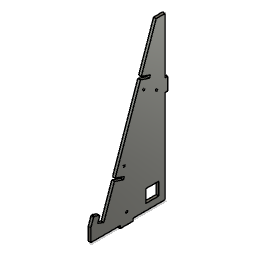
tablet_stand_R (Autodesk Fusion 360 design; units mm, degrees)
Autodesk Fusion 360 part; units mm, degrees
note: some values were not read from the file. Set by a fixed rule: the direction of a hole.
sketch "スケッチ1" plane through (0, 0, 0) normal (1, 0, 0) x (0, 0, -1)
  line L0 (-116, 0) -> (-116, 20)
  line L1 (-116, 20) -> (-111.3943, 33.2207)
  line L2 (-111.3943, 33.2207) -> (-101.951, 29.931)
  line L3 (-101.951, 29.931) -> (-105.2407, 20.4876)
  line L4 (-105.2407, 20.4876) -> (-95.7973, 17.1978)
  line L5 (-14, 252) -> (0, 252)
  line L6 (-95.7973, 17.1978) -> (-79.3485, 64.4147)
  line L7 (-79.3485, 64.4147) -> (-65.1834, 59.4801)
  line L8 (-65.1834, 59.4801) -> (-63.8675, 63.2574)
  line L9 (-63.8675, 63.2574) -> (-78.0326, 68.1921)
  line L10 (-78.0326, 68.1921) -> (-38.5555, 181.5127)
  line L11 (-38.5555, 181.5127) -> (-24.3904, 176.578)
  line L12 (-24.3904, 176.578) -> (-23.0745, 180.3554)
  line L13 (-23.0745, 180.3554) -> (-37.2396, 185.29)
  line L14 (-37.2396, 185.29) -> (-14, 252)
  line L15 (-116, 0) -> (-70, 0)
  line L16 (-70, 0) -> (-70, -4)
  line L17 (-70, -4) -> (-50, -4)
  line L18 (-50, -4) -> (-50, 0)
  line L19 (-50, 0) -> (0, 0)
  line L20 (0, 252) -> (0, 165)
  line L21 (0, 165) -> (4, 165)
  line L22 (4, 165) -> (4, 145)
  line L23 (4, 145) -> (0, 145)
  line L24 (0, 145) -> (0, 0)
  line L25 (4, 155) -> (-13.5, 155)
  line L26 (-60, -4) -> (-60, 13.5)
  line L27 (-64.1481, 77.6509) -> (-33.5533, 165.4743)
  line L28 (-10, 10) -> (-30, 10)
  line L29 (-30, 10) -> (-30, 30)
  line L30 (-30, 30) -> (-10, 30)
  line L31 (-10, 30) -> (-10, 10)
  dimension "d1" = 116
  dimension "d2" = 20
  dimension "d3" = 14
  dimension "d4" = 10
  dimension "d5" = 10
  dimension "d6" = 10
  dimension "d9" = 14
  dimension "d11" = 252
  dimension "d12" = 248.642
  dimension "d13" = 4
  dimension "d14" = 4
  dimension "d15" = 120
  dimension "d16" = 50
  dimension "d17" = 15
  dimension "d18" = 20
  dimension "d19" = 4
  dimension "d20" = 50
  dimension "d21" = 4
  dimension "d22" = 20
  dimension "d23" = 145
  dimension "d24" = 17.5
  dimension "d25" = 17.5
  dimension "d31" = 10
  dimension "d32" = 13.5
  dimension "d33" = 13.5
  dimension "d36" = 10
  dimension "d37" = 20
  dimension "d38" = 20
  dimension "d39" = 10
  constraint perpendicular L2 L3
  constraint perpendicular L1 L4
  constraint perpendicular L1 L2
  constraint perpendicular L4 L6
  constraint perpendicular L6 L7
  constraint perpendicular L7 L8
  constraint perpendicular L8 L9
  constraint perpendicular L8 L11
  constraint perpendicular L11 L12
  constraint perpendicular L12 L13
  constraint collinear L10 L14
  constraint collinear L6 L10
  constraint collinear L8 L12
  constraint perpendicular L0 L15
  constraint perpendicular L15 L16
  constraint perpendicular L0 L17
  constraint perpendicular L17 L18
  constraint coincident L19.end L24.end
  constraint perpendicular L18 L19
  constraint collinear L15 L19
  constraint horizontal L15
  constraint vertical L20
  constraint perpendicular L20 L21
  constraint perpendicular L21 L22
  constraint perpendicular L20 L23
  constraint perpendicular L19 L24
  constraint collinear L20 L24
  constraint midpoint L22 L25.start
  constraint perpendicular L22 L25
  constraint midpoint L17 L26.start
  constraint perpendicular L17 L26
  constraint parallel L10 L27
  constraint perpendicular L5 L20
  constraint horizontal L28
  constraint vertical L29
  constraint horizontal L30
  constraint vertical L31
  measures "d1" distance of L19.end L0.start
  measures "d2" distance of L0.start L0.end
  measures "d3" distance of L0.end L1.end
  measures "d4" distance of L1.end L2.end
  measures "d5" distance of L2.end L3.end
  measures "d6" distance of L3.end L4.end
  measures "d9" distance of L5.start L5.end
  measures "d11" distance of L19.end L5.end
  measures "d12" distance of L4.end L5.start
  measures "d13" distance of L11 L13
  measures "d14" distance of L7 L9
  measures "d15" distance of L9 L11
  measures "d16" distance of L4.end L6.end
  measures "d17" distance of L6.end L7.end
  measures "d18" distance of L16.end L17.end
  measures "d19" distance of L17.end L18.end
  measures "d20" distance of L18.end L19.end
  measures "d21" distance of L20.end L21.end
  measures "d22" distance of L21.end L22.end
  measures "d23" distance of L19.end L23.end
  measures "d24" distance of L25.start L25.end
  measures "d25" distance of L26.start L26.end
  measures "d31" distance of L10 L27
  measures "d32" distance of L11 L27.end
  measures "d33" distance of L9 L27.start
  measures "d36" distance of L19.end L28
  measures "d37" distance of L28.start L30.end
  measures "d38" distance of L28.start L28.end
  measures "d39" distance of L19.end L31
extrude "押し出し1" add sketch "スケッチ1" along normal blind 4
hole "穴1" at (0, 155, 13.5) at (0, 13.5, 60) at (0, 77.6509, 64.1481) at (0, 165.4743, 33.5533) direction (1, 0, 0) diameter 3.2 end through all
fillet "フィレット1" radius 1 2 edges at (2, 29.931, 101.951) (2, 33.2207, 111.3943)
